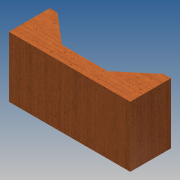
# Autodesk Inventor part: poleStandBracket
Saved by Autodesk Inventor 2013 SP2 (Build 170200200, 200)
## iProperties
Created: 2013-12-04
Part Number: poleStandBracket
Material: Wood (Cherry)
Document SubType Name: Modeling
Designer: Dave
Mass: 428.112 g
Surface Area: 751.995 cm^2
Volume: 856.224 cm^3
Density: 0.5 g/cm^3
Author: Dave
Autodesk Inventor part; units mm, degrees
ref_plane "YZ Plane" through (0, 0, 0) normal (1, 0, 0) x (0, 1, 0)
ref_plane "XZ Plane" through (0, 0, 0) normal (0, 1, 0) x (-1, 0, 0)
ref_plane "XY Plane" through (0, 0, 0) normal (0, 0, 1) x (1, 0, 0)
sketch "Sketch1" plane through (0, 0, 0) normal (0, 1, 0) x (-1, 0, 0)
  line L0 (0, 0) -> (-203.2, 0)
  circle A0 centre (-101.6, -127) radius 101.6 construction
  line L1 (-101.6, -25.4) -> (-139.7, -25.4)
  line L2 (-139.7, -25.4) -> (-190.5, -68.2625)
  line L3 (-190.5, -68.2625) -> (-203.2, -68.2625)
  line L4 (-203.2, -68.2625) -> (-203.2, 0)
  line L5 (-101.6, 0) -> (-101.6, -15.875) construction
  line L6 (-101.6, -25.4) -> (-63.5, -25.4)
  line L7 (-63.5, -25.4) -> (-12.7, -68.2625)
  line L8 (-12.7, -68.2625) -> (0, -68.2625)
  line L9 (0, -68.2625) -> (0, 0) construction
  line L10 (0, -68.2625) -> (0, 0)
  dimension "d5" = 203.2
  dimension "d4" = 203.2
  dimension "d6" = 127
  dimension "d7" = 38.1
  constraints: 22 end point, 3 parallel, 3 symmetric about line, 2 horizontal, 1 collinear, 1 midpoint, 1 vertical alignment, 2 other
  measures "d4" distance of L0.start L0.end
  measures "d6" distance from line of L0 point (-101.6, -127)
  measures "d7" distance of L1.start L1.end
extrude "Extrusion1" add sketch "Sketch1" along normal blind 101.6
body "Solid1"
